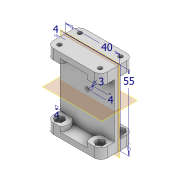
# Autodesk Inventor part: DriverHolderInside
Saved by Autodesk Inventor 2022 (Build 260153000, 153)
## iProperties
Created: 2022-11-10
Part Number: DriverHolderInside
Material: Generic
Document SubType Name: Modeling
Designer: MVeszpremi
Density: 1 g/cm^3
Appearance: Default
Author: MVeszpremi
Autodesk Inventor part; units mm, degrees
ref_plane "YZ Plane" through (0, 0, 0) normal (1, 0, 0) x (0, 1, 0)
ref_plane "XZ Plane" through (0, 0, 0) normal (0, 1, 0) x (-1, 0, 0)
ref_plane "XY Plane" through (0, 0, 0) normal (0, 0, 1) x (1, 0, 0)
sketch "Sketch4" plane through (0, 0, 0) normal (0, 0, 1) x (1, 0, 0)
  line L0 (-20, -27.5) -> (20, -27.5)
  line L1 (20, -27.5) -> (20, 27.5)
  line L2 (20, 27.5) -> (-20, 27.5)
  line L3 (-20, 27.5) -> (-20, -27.5)
  line L4 (-20, -27.5) -> (20, 27.5) construction
  line L5 (20, -27.5) -> (-20, 27.5) construction
  circle A0 centre (0, 4) radius 1.5
  line L6 (-20, 27.5) -> (20, 27.5)
  line L7 (20, 27.5) -> (20, 23.5)
  line L8 (20, 23.5) -> (-20, 23.5)
  line L9 (-20, 23.5) -> (-20, 27.5)
  line L10 (-20, -27.5) -> (20, -27.5)
  line L11 (20, -27.5) -> (20, -23.5)
  line L12 (20, -23.5) -> (-20, -23.5)
  line L13 (-20, -23.5) -> (-20, -27.5)
  point P0 (0, 0)
  point P1 (-20, -23.5)
  dimension "d33" = 55
  dimension "d34" = 40
  dimension "d35" = 3
  dimension "d36" = 4
  dimension "d37" = 4
  dimension "d38" = 4
  constraints: 28 end point, 6 parallel, 3 horizontal, 3 perpendicular, 2 midpoint, 2 point on line, 1 centre point
  measures "d33" distance of L0.end L1.end
  measures "d34" distance of L1.end L2.end
  measures "d35" diameter of A0
  measures "d36" distance of point (0, 0) A0.centre
  measures "d37" distance between parallel lines of L2 L8
  measures "d38" distance between parallel lines of L0 L12
extrude "Extrusion4" add sketch "Sketch4" along normal blind 4 contours L3 L8 L1 L12
extrude "Extrusion5" add sketch "Sketch4" along normal blind 14 and the other way blind 10 contours L3 L12 L1 L0 | L3 L2 L1 L8
sketch "Sketch5" plane through (-20, -23.5, 4) normal (0, 1, 0) x (1, 0, 0)
  line L0 (0, 14) -> (0, -10) projected
  line L1 (0, 2) -> (40, 2)
  line L2 (40, 14) -> (40, -10) projected
  line L3 (5, -5.5) -> (35, -5.5)
  line L4 (35, -5.5) -> (35, 9.5)
  line L5 (35, 9.5) -> (5, 9.5)
  line L6 (5, 9.5) -> (5, -5.5)
  line L7 (5, -5.5) -> (35, 9.5) construction
  line L8 (35, -5.5) -> (5, 9.5) construction
  circle A0 centre (5, 9.5) radius 1.5
  circle A1 centre (35, 9.5) radius 1.5
  circle A2 centre (35, -5.5) radius 1.5
  circle A3 centre (5, -5.5) radius 1.5
  point P0 (20, 4)
  point P1 (20, 2)
  dimension "d45" = 15
  dimension "d46" = 30
  dimension "d47" = 3
  dimension "d48" = 3
  dimension "d49" = 3
  dimension "d50" = 3
  constraints: 14 end point, 5 midpoint, 4 centre point, 4 coincident, 2 parallel, 1 horizontal, 1 perpendicular
  measures "d45" distance of L3.end L4.end
  measures "d46" distance of L4.end L5.end
  measures "d47" diameter of A0
  measures "d48" diameter of A3
  measures "d49" diameter of A2
  measures "d50" diameter of A1
extrude "Extrusion6" cut sketch "Sketch5" against normal blind 14 contours A0 L5 L6 | L6 L5 A0 | A3 L3 L6 | L6 L3 A3 | A2 L3 L4 | L4 L3 A2 | A1 L5 L4 | L4 L5 A1
sketch "Sketch6" plane through (-20, -23.5, 4) normal (0, 1, 0) x (1, 0, 0)
  circle A0 centre (5, -5.5) radius 1.5 projected
  line L0 (5, -2.0359) -> (8, -3.7679)
  line L1 (8, -3.7679) -> (8, -7.2321)
  line L2 (8, -7.2321) -> (5, -8.9641)
  line L3 (5, -8.9641) -> (2, -7.2321)
  line L4 (2, -7.2321) -> (2, -3.7679)
  line L5 (2, -3.7679) -> (5, -2.0359)
  circle A1 centre (35, -5.5) radius 1.5 projected
  line L6 (35, -8.9641) -> (32, -7.2321)
  line L7 (32, -7.2321) -> (32, -3.7679)
  line L8 (32, -3.7679) -> (35, -2.0359)
  line L9 (35, -2.0359) -> (38, -3.7679)
  line L10 (38, -3.7679) -> (38, -7.2321)
  line L11 (38, -7.2321) -> (35, -8.9641)
  circle A2 centre (5, -5.5) radius 1.5 projected
  line L12 (40, -10) -> (0, -10) projected
  circle A3 centre (5, -5.5) radius 6.7268
  circle A4 centre (35, -5.5) radius 1.5 projected
  line L13 (40, 14) -> (40, -10) projected
  circle A5 centre (35, -5.5) radius 6.7268
  circle A6 centre (35, -5.5) radius 1.5 projected
  circle A7 centre (5, -5.5) radius 1.5 projected
  line L14 (0, 0) -> (40, 0) projected
  line L15 (0, -10) -> (0, 0) projected
  line L16 (40, -10) -> (0, -10) projected
  line L17 (40, 0) -> (40, -10) projected
  point P0 (20, 4)
  point P1 (38.873, 0)
  point P2 (31.127, 0)
  point P3 (30, -10)
  point P4 (40, -1)
  point P5 (0, -1)
  point P6 (0, -10)
  point P7 (10, -10)
  point P8 (8.873, 0)
  point P9 (1.127, 0)
  dimension "d53" = 6
  dimension "d54" = 6
  constraints: 24 end point, 4 coincident, 32 other
  measures "d53" distance between parallel lines of L1 L4
  measures "d54" distance between parallel lines of L7 L10
extrude "Extrusion7" add sketch "Sketch6" along normal blind 3.5 contours L12 A5 L14 L13 | A5 L14 L13 | L12 L15 A3 L14 | L15 L14 A3
ref_plane "Work Plane1" through (0, 0, 2) normal (0, 0, 1) x (1, 0, 0)
mirror "Mirror1" about plane through (0, 0, 2) normal (0, 0, 1) of "Extrusion7"
ref_plane "Work Plane2" through (-11.127, 0, 0) normal (0, 1, 0) x (1, 0, 0)
mirror "Mirror2" about plane through (-11.127, 0, 0) normal (0, 1, 0) of "Extrusion7", "Mirror1", "Extrusion6"
fillet "Fillet2" radius 5 4 edges at (-20, 23.75, 14) (-20, 23.75, -10) (20, 23.75, 14) (20, 23.75, -10)
fillet "Fillet3" radius 5 4 edges at (-20, -23.75, 14) (-20, -23.75, -10) (20, -23.75, 14) (20, -23.75, -10)
body "Solid2"
